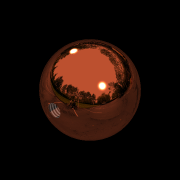
# Autodesk Inventor part: ShiftBall
Saved by Autodesk Inventor 2022 (Build 260153000, 153)
## iProperties
Created: 2020-12-29
Part Number: ShiftBall
Material: Generic
Document SubType Name: Modeling
Designer: jdski
Density: 1 g/cm^3
Appearance: Default
Author: jdski
Autodesk Inventor part; units mm, degrees
ref_plane "YZ Plane" through (0, 0, 0) normal (1, 0, 0) x (0, 1, 0)
ref_plane "XZ Plane" through (0, 0, 0) normal (0, 1, 0) x (-1, 0, 0)
ref_plane "XY Plane" through (0, 0, 0) normal (0, 0, 1) x (1, 0, 0)
sketch "Sketch1" plane through (0, 0, 0) normal (0, 0, 1) x (1, 0, 0)
  arc A0 (12.7, 0) -> (-12.7, 0) centre (0, 0) ccw
  line L0 (0, 0) -> (12.7, 0) construction
  line L1 (0, 0) -> (12.7, 0) construction
  line L2 (0, 0) -> (-12.7, 0) construction
  line L3 (-12.7, 0) -> (12.7, 0)
  circle A1 centre (0, 0) radius 2.0828
  dimension "d0" = 12.7
  dimension "d1" = 0
  dimension "d2" = 180
  dimension "d4" = 4.1656
  constraints: 8 end point, 2 centre point, 2 coincident, 2 point on circle, 1 collinear, 1 horizontal
  measures "d0" radius of A0
  measures "d1" distance between parallel lines of L0 L1
  measures "d2" angle of L2 L0
  measures "d4" diameter of A1
revolve "Revolution1" add sketch "Sketch1" angle 360 about axis through (-12.7, 0, 0) along (1, 0, 0) picked at (0.5197, 0.4604) contours L3 A1 A0 | L3 A1
extrude "Extrusion3" cut sketch "Sketch1" along normal mid plane 25.4 contours A1 L3 | L3 A1
thread "Thread2" size "8-32 UNC" class "2B" standard "ANSI Unified Screw Threads" length 25.4
body "Solid1"
